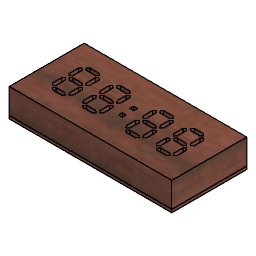
7-segment-display-colorized (Autodesk Fusion 360 design; units mm, degrees)
part number: 2025-10-20-08-46-35-604
Autodesk Fusion 360 part; units mm, degrees
note: some values were not read from the file. Chosen so that the rebuilt part matches the saved one: which face or edge a step refers to.
box "BoxPrimitive1" add length 60 width 130 height 20 placed x (0, 1, 0) y (-1, 0, 0) z (0, 0, 1) at (30, -50, 0) makes body 1
box "BoxPrimitive2" add length 50 width 120 height 10 placed x (0, 1, 0) y (-1, 0, 0) z (0, 0, 1) at (25, -45, 0) separate body makes body 2
move_body "Move1" bodies 2 to x (1, 0, 0) y (0, 1, 0) z (0, 0, 1) at (0, 0, 5)
sketch "Sketch6" plane through (0, 0, 0) normal (0, 0, 1) x (1, 0, 0)
  line L0 (0, 102.5) -> (0, 105)
  line L1 (0, 105) -> (0.5, 105.5)
  line L2 (0.5, 105.5) -> (1, 105)
  line L3 (1, 105) -> (1, 102.5)
  line L4 (1, 102.5) -> (0.5, 102)
  line L5 (0.5, 102) -> (0, 102.5)
  line L6 (1, 101.5) -> (1.5, 102)
  line L7 (1.5, 102) -> (4, 102)
  line L8 (4, 102) -> (4.5, 101.5)
  line L9 (4.5, 101.5) -> (4, 101)
  line L10 (4, 101) -> (1.5, 101)
  line L11 (1.5, 101) -> (1, 101.5)
  line L12 (4.5, 102.5) -> (4.5, 105)
  line L13 (4.5, 105) -> (5, 105.5)
  line L14 (5, 105.5) -> (5.5001, 105)
  line L15 (5.5001, 105) -> (5.5001, 102.5)
  line L16 (5.5001, 102.5) -> (5, 101.9999)
  line L17 (5, 101.9999) -> (4.5, 102.5)
  line L18 (1.5, 105.5) -> (1, 106)
  line L19 (1, 106) -> (1.5, 106.5)
  line L20 (1.5, 106.5) -> (4, 106.5)
  line L21 (4, 106.5) -> (4.5, 106)
  line L22 (4.5, 106) -> (4, 105.5)
  line L23 (4, 105.5) -> (1.5, 105.5)
  line L24 (0.5, 106.5) -> (1, 107)
  line L25 (1, 107) -> (1, 109.5)
  line L26 (1, 109.5) -> (0.5, 110)
  line L27 (0.5, 110) -> (0, 109.5)
  line L28 (0, 109.5) -> (0, 107)
  line L29 (0, 107) -> (0.5, 106.5)
  line L30 (5, 106.5) -> (4.5, 107)
  line L31 (4.5, 107) -> (4.5, 109.5)
  line L32 (4.5, 109.5) -> (5, 110)
  line L33 (5, 110) -> (5.5, 109.5)
  line L34 (5.5, 109.5) -> (5.5, 107)
  line L35 (5.5, 107) -> (5, 106.5)
  line L36 (4, 110) -> (4.5, 110.5)
  line L37 (4.5, 110.5) -> (4, 111)
  line L38 (4, 111) -> (1.5, 111)
  line L39 (1.5, 111) -> (1, 110.5)
  line L40 (1, 110.5) -> (1.5, 110)
  line L41 (1.5, 110) -> (4, 110)
  constraint vertical L0
  constraint perpendicular L1 L2
  constraint parallel L0 L3
  constraint perpendicular L2 L4
  constraint perpendicular L5 L6
  constraint horizontal L7
  constraint perpendicular L6 L8
  constraint parallel L7 L10
  constraint perpendicular L13 L14
  constraint parallel L12 L15
  constraint perpendicular L14 L16
  constraint perpendicular L18 L19
  constraint horizontal L20
  constraint perpendicular L19 L21
  constraint perpendicular L18 L22
  constraint parallel L20 L23
  constraint perpendicular L18 L24
  constraint perpendicular L23 L25
  constraint perpendicular L24 L26
  constraint perpendicular L26 L27
  constraint parallel L25 L28
  constraint perpendicular L27 L29
  constraint perpendicular L24 L30
  constraint parallel L28 L31
  constraint perpendicular L30 L32
  constraint perpendicular L32 L33
  constraint parallel L31 L34
  constraint perpendicular L30 L35
  constraint perpendicular L30 L36
  constraint perpendicular L36 L37
  constraint horizontal L38
  constraint perpendicular L37 L39
  constraint perpendicular L39 L40
  constraint parallel L38 L41
extrude "Extrude3" add sketch "Sketch6" along normal blind 5 separate body makes body 3 at (1, 104.1667, 1.6667) makes body 4 at (2.3333, 110, 1.6667) makes body 5 at (3.1667, 105.5, 1.6667) makes body 6 at (4.5, 103.3333, 1.6667) makes body 7 at (0, 108.6667, 1.6667) makes body 8 at (4.5, 107.8333, 1.6667) makes body 9 at (3.1667, 101, 1.6667)
move_body "Move10" bodies 4 8 6 3 5 9 7 to x (1, 0, 0) y (0, 1, 0) z (0, 0, 1) at (-96.5, -96, 15)
move_body "Move11" bodies 5 4 7 8 3 6 9 to x (1, 0, 0) y (0, 1, 0) z (0, 0, 1) at (20, 0, 0)
scale "Scale1" factors (3, 3, 1) about (-72.5, 5, 15) bodies 3 5 7 4 8 6 9
move_body "Move12" bodies 6 8 9 4 7 5 3 to x (1, 0, 0) y (0, 1, 0) z (0, 0, 1) at (-0.5, -40, 0)
copy_body "CopyPasteBodies6" bodies 6 3 5 4 9 7 8 makes body 10 makes body 11 makes body 12 makes body 13 makes body 14 makes body 15 makes body 16
move_body "Move14" bodies 10 11 12 13 14 15 16 to x (1, 0, 0) y (0, 1, 0) z (0, 0, 1) at (24.5, 0, 0)
copy_body "CopyPasteBodies7" bodies 6 3 5 4 9 7 8 makes body 17 makes body 18 makes body 19 makes body 20 makes body 21 makes body 22 makes body 23
move_body "Move15" bodies 17 18 19 20 21 22 23 to x (1, 0, 0) y (0, 1, 0) z (0, 0, 1) at (59, 0, 0)
copy_body "CopyPasteBodies8" bodies 6 3 5 4 9 7 8 makes body 24 makes body 25 makes body 26 makes body 27 makes body 28 makes body 29 makes body 30
move_body "Move16" bodies 24 25 26 27 28 29 30 to x (1, 0, 0) y (0, 1, 0) z (0, 0, 1) at (83.5, 0, 0)
sketch "Sketch7" plane through (0, 0, 0) normal (0, 0, 1) x (1, 0, 0)
  line L0 (0, 100) -> (3, 100)
  line L1 (3, 100) -> (3, 103)
  line L2 (3, 103) -> (0, 103)
  line L3 (0, 103) -> (0, 100)
  line L4 (0, 109) -> (3, 109)
  line L5 (3, 109) -> (3, 112)
  line L6 (3, 112) -> (0, 112)
  line L7 (0, 112) -> (0, 109)
  constraint horizontal L0
  constraint vertical L1
  constraint horizontal L2
  constraint vertical L3
  constraint horizontal L4
  constraint vertical L5
  constraint horizontal L6
  constraint vertical L7
extrude "Extrude4" add sketch "Sketch7" along normal blind 5 separate body makes body 31 at (0, 111, 1.6667) makes body 32 at (0, 102, 1.6667)
move_body "Move17" bodies 31 32 to x (1, 0, 0) y (0, 1, 0) z (0, 0, 1) at (-43.9998, -123.0001, 15)
move_body "Move18" bodies 31 32 to x (1, 0, 0) y (0, 1, 0) z (0, 0, 1) at (7.5, -3, 0)
combine "Combine3" operation add target body 2 tool bodies 13 32 23 17 14 4 28 24 20 3 11 31 8 6 9 15 7 10 5 19 30 21 25 27 12 22 29 18 26 16 keep tools
extrude "Extrude5" add 1 faces at (-55, -28.3333, 5) along direction (0, 0, -1) blind 5 on bodies 2 bodies 2
combine "Combine4" operation cut target body 1 tool bodies 2
copy_body "CopyPasteBodies9" bodies 3 4 5 6 7 8 9 makes body 33 makes body 34 makes body 35 makes body 36 makes body 37 makes body 38 makes body 39
move_body "Move20" bodies 33 34 35 36 37 38 39 to x (1, 0, 0) y (0, 1, 0) z (0, 0, 1) at (-50, 0, 0)
copy_body "CopyPasteBodies10" bodies 33 34 35 36 37 38 39 makes body 40 makes body 41 makes body 42 makes body 43 makes body 44 makes body 45 makes body 46
move_face "OffsetFaces1" offset 0.5 56 faces at (-131.5, -7, 16.6667) (-122.5, -7.5, 16.6667) (-128, -8, 16.6667) (-128, -7, 15) (-131, -5.5, 16.6667) (-122, -6, 16.6667) (-125.5, -5, 16.6667) (-128, -7, 20) (-128, -34, 15) (-128, -34, 20) (-122.5, -32.5, 16.6667) (-131.5, -33, 16.6667) (-131, -34.5, 16.6667) (-122, -34, 16.6667) (-128, -32, 16.6667) (-125.5, -35, 16.6667) (-134, -8.5, 16.6667) (-134.5, -17.5, 16.6667) (-133, -18, 16.6667) (-134, -12, 15) (-132.5, -9, 16.6667) (-132, -14.5, 16.6667) (-135, -12, 16.6667) (-134, -12, 20) (-120.5, -12, 15) (-120.5, -12, 20) (-121, -9, 16.6667) (-119, -17.5, 16.6667) (-119.5, -8.5, 16.6667) (-120.5, -18, 16.6667) (-121.5, -14.5, 16.6667) (-118.5, -12, 16.6667) (-122, -20.5, 16.6667) (-122.5, -19, 16.6667) (-125.5, -20.5, 20) (-131, -21, 16.6667) (-125.5, -20.5, 15) (-125.5, -21.5, 16.6667) (-131.5, -19.5, 16.6667) (-128, -18.5, 16.6667) (-118.9999, -22.5001, 18.3333) (-118.9999, -31.0001, 16.6667) (-120.4999, -25.5001, 15) (-121.5, -28, 16.6667) (-120.5, -31.5002, 16.6667) (-121, -22.5001, 16.6667) (-118.4998, -25.5001, 16.6667) (-120.4999, -25.5001, 20) (-133, -22, 16.6667) (-133, -28, 15) (-132.5, -31, 16.6667) (-135, -28, 18.3333) (-132, -25.5, 16.6667) (-133, -28, 20) (-134, -31.5, 16.6667) (-134.5, -22.5, 16.6667) on bodies 40 41 42 43 44 45 46
extrude "Extrude6" add 7 faces at (-128, -34, 15) (-133, -28, 15) (-125.5, -20.5, 15) (-120.4999, -25.5001, 15) (-120.5, -12, 15) (-128, -7, 15) (-134, -12, 15) along direction (0, 0, -1) blind 0.5 on bodies 33 34 35 36 37 38 39 bodies 39 33 34 35 36 37 38
extrude "Extrude7" add 7 faces at (-128, -34, 20) (-120.4999, -25.5001, 20) (-125.5, -20.5, 20) (-133, -28, 20) (-134, -12, 20) (-128, -7, 20) (-120.5, -12, 20) along direction (0, 0, 1) blind 0.5 on bodies 33 34 35 36 37 38 39 bodies 39 33 34 35 36 37 38
combine "Combine5" operation cut target body 46 tool bodies 39
combine "Combine6" operation cut target body 43 tool bodies 36
combine "Combine7" operation cut target body 42 tool bodies 35
combine "Combine8" operation cut target body 40 tool bodies 33
combine "Combine9" operation cut target body 45 tool bodies 38
combine "Combine10" operation cut target body 44 tool bodies 37
combine "Combine11" operation cut target body 41 tool bodies 34
copy_body "CopyPasteBodies12" bodies 40 41 42 43 44 45 46 makes body 47 makes body 48 makes body 49 makes body 50 makes body 51 makes body 52 makes body 53
move_body "Move22" bodies 47 48 49 50 51 52 53 to x (1, 0, 0) y (0, 1, 0) z (0, 0, 1) at (50, 0, -5.5)
copy_body "CopyPasteBodies14" bodies 40 41 42 43 44 45 46 makes body 54 makes body 55 makes body 56 makes body 57 makes body 58 makes body 59 makes body 60
copy_body "CopyPasteBodies15" bodies 40 41 42 43 44 45 46 makes body 61 makes body 62 makes body 63 makes body 64 makes body 65 makes body 66 makes body 67
copy_body "CopyPasteBodies16" bodies 40 41 42 43 44 45 46 makes body 68 makes body 69 makes body 70 makes body 71 makes body 72 makes body 73 makes body 74
move_body "Move23" bodies 58 59 56 54 60 57 55 to x (1, 0, 0) y (0, 1, 0) z (0, 0, 1) at (74.5, 0, -5.5)
move_body "Move24" bodies 66 62 64 65 63 67 61 to x (1, 0, 0) y (0, 1, 0) z (0, 0, 1) at (109, 0, -5.5)
move_body "Move25" bodies 74 73 70 71 69 72 68 to x (1, 0, 0) y (0, 1, 0) z (0, 0, 1) at (133.5, 0, -5.5)
copy_body "CopyPasteBodies17" bodies 31 32 makes body 75 makes body 76
move_body "Move26" bodies 75 76 to x (1, 0, 0) y (0, 1, 0) z (0, 0, 1) at (100, 0, 0)
copy_body "CopyPasteBodies18" bodies 75 76 makes body 77 makes body 78
move_face "OffsetFaces2" offset 0.5 12 faces at (64.5002, -15.0001, 15) (66.5002, -16.0001, 16.6667) (64.5002, -15.0001, 20) (63.5002, -15.0001, 16.6667) (65.5002, -14.0001, 16.6667) (64.5002, -17.0001, 16.6667) (66.5002, -25.0001, 16.6667) (64.5002, -24.0001, 20) (64.5002, -26.0001, 16.6667) (63.5002, -24.0001, 16.6667) (65.5002, -23.0001, 16.6667) (64.5002, -24.0001, 15) on bodies 77 78
extrude "Extrude8" add 1 faces at (64.5002, -24.0001, 15) along direction (0, 0, -1) blind 0.5 on bodies 76 bodies 76
extrude "Extrude9" add 1 faces at (64.5002, -15.0001, 15) along direction (0, 0, -1) blind 0.5 on bodies 75 bodies 75
extrude "Extrude10" add 1 faces at (64.5002, -15.0001, 20) along direction (0, 0, 1) blind 0.5 on bodies 75 bodies 75
extrude "Extrude11" add 1 faces at (64.5002, -24.0001, 20) along direction (0, 0, 1) blind 0.5 on bodies 76 bodies 76
combine "Combine12" operation cut target body 77 tool bodies 75
combine "Combine13" operation cut target body 78 tool bodies 76
move_body "Move27" bodies 78 77 to x (1, 0, 0) y (0, 1, 0) z (0, 0, 1) at (-100, 0, -5.5)
box "BoxPrimitive3" add length 60 width 130 height 2.5 placed x (0, 1, 0) y (-1, 0, 0) z (0, 0, 1) at (170, -50, 0) separate body makes body 79
box "BoxPrimitive4" add length 6 width 2 height 0.5 placed x (0, 1, 0) y (-1, 0, 0) z (0, 0, 1) at (42, 15, 0) separate body makes body 80
box "BoxPrimitive5" add length 1 width 1 height 0.5 placed x (0, 1, 0) y (-1, 0, 0) z (0, 0, 1) at (41.5, 17.5, 0.5) separate body makes body 81
box "BoxPrimitive6" add length 0.5 width 0.25 height 0.25 placed x (0, 1, 0) y (-1, 0, 0) z (0, 0, 1) at (40.75, 15, 0.5) separate body makes body 82
copy_body "CopyPasteBodies19" bodies 82 makes body 83
move_body "Move28" bodies 83 to x (1, 0, 0) y (0, 1, 0) z (0, 0, 1) at (0.375, 0, 0)
copy_body "CopyPasteBodies20" bodies 82 makes body 84
move_body "Move29" bodies 84 to x (1, 0, 0) y (0, 1, 0) z (0, 0, 1) at (0.75, 0, 0)
copy_body "CopyPasteBodies21" bodies 82 83 84 makes body 85 makes body 86 makes body 87
move_body "Move30" bodies 85 86 87 to x (1, 0, 0) y (0, 1, 0) z (0, 0, 1) at (0, 5.5, 0)
copy_body "CopyPasteBodies22" bodies 80 makes body 88
copy_body "CopyPasteBodies23" bodies 81 makes body 89
move_body "Move31" bodies 89 to x (1, 0, 0) y (0, 1, 0) z (0, 0, 1) at (0, 1.25, 0)
move_body "Move32" bodies 81 to x (1, 0, 0) y (0, 1, 0) z (0, 0, 1) at (0, -1.25, 0)
move_body "Move33" bodies 85 88 86 80 83 84 81 82 89 87 to x (1, 0, 0) y (0, 1, 0) z (0, 0, 1) at (0, -5, 2.5)
move_body "Move34" bodies 85 88 86 80 83 84 81 82 89 87 to x (1, 0, 0) y (0, 1, 0) z (0, 0, 1) at (15.5, -26.25, 0)
copy_body "CopyPasteBodies25" bodies 80 81 82 83 84 85 86 87 88 89 makes body 90 makes body 91 makes body 92 makes body 93 makes body 94 makes body 95 makes body 96 makes body 97 makes body 98 makes body 99
move_body "Move36" bodies 90 91 92 93 94 95 96 97 98 99 to x (1, 0, 0) y (0, 1, 0) z (0, 0, 1) at (13.5, 0, 0)
copy_body "CopyPasteBodies26" bodies 80 81 82 83 84 85 86 87 88 89 90 91 92 93 94 95 96 97 98 99 makes body 100 makes body 101 makes body 102 makes body 103 makes body 104 makes body 105 makes body 106 makes body 107 makes body 108 makes body 109 makes body 110 makes body 111 makes body 112 makes body 113 makes body 114 makes body 115 makes body 116 makes body 117 makes body 118 makes body 119
move_body "Move37" bodies 100 101 102 103 104 105 106 107 108 109 110 111 112 113 114 115 116 117 118 119 to x (1, 0, 0) y (0, 1, 0) z (0, 0, 1) at (0, -13.5, 0)
copy_body "CopyPasteBodies28" bodies 80 81 82 83 84 85 86 87 88 89 makes body 120 makes body 121 makes body 122 makes body 123 makes body 124 makes body 125 makes body 126 makes body 127 makes body 128 makes body 129
move_body "Move40" bodies 120 121 122 123 124 125 126 127 128 129 to x (0, -1, 0) y (1, 0, 0) z (0, 0, 1) at (71.75, 39.25, 0)
move_body "Move41" bodies 120 121 122 123 124 125 126 127 128 129 to x (1, 0, 0) y (0, 1, 0) z (0, 0, 1) at (4.75, 10.75, 0)
copy_body "CopyPasteBodies29" bodies 120 121 122 123 124 125 126 127 128 129 makes body 130 makes body 131 makes body 132 makes body 133 makes body 134 makes body 135 makes body 136 makes body 137 makes body 138 makes body 139
move_body "Move43" bodies 130 131 132 133 134 135 136 137 138 139 to x (1, 0, 0) y (0, 1, 0) z (0, 0, 1) at (0, -13.5, 0)
copy_body "CopyPasteBodies30" bodies 120 121 122 123 124 125 126 127 128 129 makes body 140 makes body 141 makes body 142 makes body 143 makes body 144 makes body 145 makes body 146 makes body 147 makes body 148 makes body 149
move_body "Move44" bodies 140 141 142 143 144 145 146 147 148 149 to x (1, 0, 0) y (0, 1, 0) z (0, 0, 1) at (0, -27, 0)
copy_body "CopyPasteBodies31" bodies 80 81 82 83 84 85 86 87 88 89 90 91 92 93 94 95 96 97 98 99 100 101 102 103 104 105 106 107 108 109 110 111 112 113 114 115 116 117 118 119 120 121 122 123 124 125 126 127 128 129 130 131 132 133 134 135 136 137 138 139 140 141 142 143 144 145 146 147 148 149 makes body 150 makes body 151 makes body 152 makes body 153 makes body 154 makes body 155 makes body 156 makes body 157 makes body 158 makes body 159 makes body 160 makes body 161 makes body 162 makes body 163 makes body 164 makes body 165 makes body 166 makes body 167 makes body 168 makes body 169 makes body 170 makes body 171 makes body 172 makes body 173 makes body 174 makes body 175 makes body 176 makes body 177 makes body 178 makes body 179 makes body 180 makes body 181 makes body 182 makes body 183 makes body 184 makes body 185 makes body 186 makes body 187 makes body 188 makes body 189 makes body 190 makes body 191 makes body 192 makes body 193 makes body 194 makes body 195 makes body 196 makes body 197 makes body 198 makes body 199 makes body 200 makes body 201 makes body 202 makes body 203 makes body 204 makes body 205 makes body 206 makes body 207 makes body 208 makes body 209 makes body 210 makes body 211 makes body 212 makes body 213 makes body 214 makes body 215 makes body 216 makes body 217 makes body 218 makes body 219
move_body "Move45" bodies 150 151 152 153 154 155 156 157 158 159 160 161 162 163 164 165 166 167 168 169 170 171 172 173 174 175 176 177 178 179 180 181 182 183 184 185 186 187 188 189 190 191 192 193 194 195 196 197 198 199 200 201 202 203 204 205 206 207 208 209 210 211 212 213 214 215 216 217 218 219 to x (1, 0, 0) y (0, 1, 0) z (0, 0, 1) at (24.5, 0, 0)
copy_body "CopyPasteBodies32" bodies 80 81 82 83 84 85 86 87 88 89 90 91 92 93 94 95 96 97 98 99 100 101 102 103 104 105 106 107 108 109 110 111 112 113 114 115 116 117 118 119 120 121 122 123 124 125 126 127 128 129 130 131 132 133 134 135 136 137 138 139 140 141 142 143 144 145 146 147 148 149 makes body 220 makes body 221 makes body 222 makes body 223 makes body 224 makes body 225 makes body 226 makes body 227 makes body 228 makes body 229 makes body 230 makes body 231 makes body 232 makes body 233 makes body 234 makes body 235 makes body 236 makes body 237 makes body 238 makes body 239 makes body 240 makes body 241 makes body 242 makes body 243 makes body 244 makes body 245 makes body 246 makes body 247 makes body 248 makes body 249 makes body 250 makes body 251 makes body 252 makes body 253 makes body 254 makes body 255 makes body 256 makes body 257 makes body 258 makes body 259 makes body 260 makes body 261 makes body 262 makes body 263 makes body 264 makes body 265 makes body 266 makes body 267 makes body 268 makes body 269 makes body 270 makes body 271 makes body 272 makes body 273 makes body 274 makes body 275 makes body 276 makes body 277 makes body 278 makes body 279 makes body 280 makes body 281 makes body 282 makes body 283 makes body 284 makes body 285 makes body 286 makes body 287 makes body 288 makes body 289
move_body "Move46" bodies 220 221 222 223 224 225 226 227 228 229 230 231 232 233 234 235 236 237 238 239 240 241 242 243 244 245 246 247 248 249 250 251 252 253 254 255 256 257 258 259 260 261 262 263 264 265 266 267 268 269 270 271 272 273 274 275 276 277 278 279 280 281 282 283 284 285 286 287 288 289 to x (1, 0, 0) y (0, 1, 0) z (0, 0, 1) at (59, 0, 0)
copy_body "CopyPasteBodies33" bodies 80 81 82 83 84 85 86 87 88 89 90 91 92 93 94 95 96 97 98 99 100 101 102 103 104 105 106 107 108 109 110 111 112 113 114 115 116 117 118 119 120 121 122 123 124 125 126 127 128 129 130 131 132 133 134 135 136 137 138 139 140 141 142 143 144 145 146 147 148 149 makes body 290 makes body 291 makes body 292 makes body 293 makes body 294 makes body 295 makes body 296 makes body 297 makes body 298 makes body 299 makes body 300 makes body 301 makes body 302 makes body 303 makes body 304 makes body 305 makes body 306 makes body 307 makes body 308 makes body 309 makes body 310 makes body 311 makes body 312 makes body 313 makes body 314 makes body 315 makes body 316 makes body 317 makes body 318 makes body 319 makes body 320 makes body 321 makes body 322 makes body 323 makes body 324 makes body 325 makes body 326 makes body 327 makes body 328 makes body 329 makes body 330 makes body 331 makes body 332 makes body 333 makes body 334 makes body 335 makes body 336 makes body 337 makes body 338 makes body 339 makes body 340 makes body 341 makes body 342 makes body 343 makes body 344 makes body 345 makes body 346 makes body 347 makes body 348 makes body 349 makes body 350 makes body 351 makes body 352 makes body 353 makes body 354 makes body 355 makes body 356 makes body 357 makes body 358 makes body 359
move_body "Move47" bodies 290 291 292 293 294 295 296 297 298 299 300 301 302 303 304 305 306 307 308 309 310 311 312 313 314 315 316 317 318 319 320 321 322 323 324 325 326 327 328 329 330 331 332 333 334 335 336 337 338 339 340 341 342 343 344 345 346 347 348 349 350 351 352 353 354 355 356 357 358 359 to x (1, 0, 0) y (0, 1, 0) z (0, 0, 1) at (83.5, 0, 0)
move_body "Move48" bodies 324 182 150 116 81 126 351 121 257 146 83 255 186 85 173 200 135 120 86 108 287 254 96 131 357 198 138 219 141 133 136 174 286 325 214 329 193 208 139 318 179 311 183 310 243 190 119 90 98 94 111 110 97 99 91 79 118 117 130 114 176 358 215 154 177 168 122 87 106 132 222 89 100 350 253 320 143 148 165 187 184 95 221 352 115 93 164 191 142 282 317 288 101 158 206 153 247 140 163 189 124 181 261 129 242 262 204 201 188 107 123 229 172 103 355 105 280 147 199 167 210 267 211 113 209 326 92 128 155 359 180 241 228 248 313 232 112 212 245 218 109 80 268 169 159 356 84 134 162 270 226 125 250 353 185 157 88 260 144 323 104 161 175 156 284 127 137 273 102 278 354 82 316 145 160 224 343 339 256 314 272 269 322 292 238 217 258 321 291 345 178 295 249 281 213 312 240 252 194 195 271 276 207 152 197 319 237 170 149 234 340 223 192 294 274 263 171 315 151 279 348 285 328 196 216 327 166 275 338 202 205 203 296 265 264 225 277 227 330 233 220 235 259 349 337 301 236 251 230 333 246 239 335 266 231 332 289 300 346 244 307 334 297 306 302 308 303 290 347 293 344 336 298 309 341 342 283 331 299 305 304 to x (1, 0, 0) y (0, 1, 0) z (0, 0, 1) at (-140, 0, -2.5)
